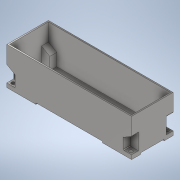
# Autodesk Inventor part: МПСТ Корпус
Saved by Autodesk Inventor 2022.1 (Build 261234020, 234B)
## iProperties
Created: 2021-11-18
Part Number: МПСТ Корпус
Material: Сталь, углеродистая
Document SubType Name: Modeling
Designer: Алексанян Г.
Density: 7.85 g/cm^3
Appearance: С умеренной полировкой
Author: Алексанян Г.
Autodesk Inventor part; units mm, degrees
ref_plane "YZ Plane" through (0, 0, 0) normal (1, 0, 0) x (0, 1, 0)
ref_plane "XZ Plane" through (0, 0, 0) normal (0, 1, 0) x (-1, 0, 0)
ref_plane "XY Plane" through (0, 0, 0) normal (0, 0, 1) x (1, 0, 0)
sketch "Эскиз1" plane through (0, 0, 0) normal (0, 1, 0) x (-1, 0, 0)
  line L0 (450, -150) -> (-450, -150)
  line L1 (-450, -150) -> (-450, 150)
  line L2 (-450, 150) -> (450, 150)
  line L3 (450, 150) -> (450, -150)
  line L4 (450, -150) -> (-450, 150) construction
  line L5 (-450, -150) -> (450, 150) construction
  point P0 (0, 0)
  dimension "d0" = 900
  dimension "d1" = 300
  constraints: 12 end point, 2 midpoint, 2 parallel, 1 horizontal, 1 perpendicular
  measures "d0" distance of L1.end L2.end
  measures "d1" distance of L0.end L1.end
extrude "Выдавливание1" add sketch "Эскиз1" against normal blind 270
sketch "Эскиз2" plane through (-450, 0, 150) normal (0, 0, 1) x (1, 0, 0)
  line L0 (210, -260) -> (690, -260)
  line L1 (690, -260) -> (690, -280)
  line L2 (690, -280) -> (210, -280)
  line L3 (210, -280) -> (210, -260)
  line L4 (900, -270) -> (0, -270) projected
  line L5 (210, -260) -> (690, -280) construction
  line L6 (690, -260) -> (210, -280) construction
  point P0 (450, 0)
  point P1 (450, -270)
  dimension "d4" = 480
  dimension "d5" = 20
  constraints: 12 end point, 3 midpoint, 2 parallel, 1 horizontal, 1 perpendicular
  measures "d4" distance of L1.end L2.end
  measures "d5" distance of L0.end L1.end
extrude "Выдавливание2" cut sketch "Эскиз2" against normal through all
sketch "Эскиз3" plane through (450, 0, 150) normal (1, 0, 0) x (0, 0, -1)
  line L0 (65, -260) -> (235, -260)
  line L1 (235, -260) -> (235, -280)
  line L2 (235, -280) -> (65, -280)
  line L3 (65, -280) -> (65, -260)
  line L4 (0, -270) -> (300, -270) projected
  line L5 (65, -260) -> (235, -280) construction
  line L6 (235, -260) -> (65, -280) construction
  point P0 (150, 0)
  point P1 (150, -270)
  dimension "d8" = 170
  dimension "d9" = 20
  constraints: 12 end point, 3 midpoint, 2 parallel, 1 horizontal, 1 perpendicular
  measures "d8" distance of L1.end L2.end
  measures "d9" distance of L0.end L1.end
extrude "Выдавливание3" cut sketch "Эскиз3" against normal through all
sketch "Эскиз4" plane through (-450, 0, 150) normal (0, 0, 1) x (1, 0, 0)
  line L0 (900, 0) -> (900, -270) projected
  line L1 (900, -240) -> (840, -240)
  line L2 (840, -240) -> (840, -160)
  line L3 (900, -110) -> (900, -240)
  line L4 (840, -160) -> (900, -125.359)
  line L5 (840, -160) -> (909.282, -160) construction
  line L6 (900, -270) -> (690, -270) projected
  point P0 (450, 0)
  point P1 (870, -240)
  dimension "d12" = 30
  dimension "d13" = 30
  dimension "d14" = 60
  dimension "d15" = 80
  constraints: 10 end point, 2 horizontal, 2 point on line, 1 equal length, 1 midpoint, 1 parallel, 1 perpendicular
  measures "d12" angle of L5 L4
  measures "d13" distance from line of L6 point (870, -240)
  measures "d14" distance between parallel lines of L2 L0
  measures "d15" distance from line of L1 L2.end
extrude "Выдавливание4" cut sketch "Эскиз4" against normal blind 50
sketch "Эскиз5" plane through (390, -240, 150) normal (0, 1, 0) x (1, 0, 0)
  line L0 (60, 50) -> (60, 0) projected
  line L1 (60, 0) -> (0, 0) projected
  point P0 (-390, 150)
  point P1 (35, 20)
  dimension "d18" = 25
  dimension "d19" = 20
  measures "d18" distance from line of L0 point (35, 20)
  measures "d19" distance from line of L1 point (35, 20)
hole "Отверстие1" at (425, -240, 130) direction (0, -1, 0) diameter 25 end through all
mirror "Зеркальное отражение1" about plane through (0, 0, 0) normal (1, 0, 0) of "Выдавливание4", "Отверстие1"
mirror "Зеркальное отражение2" about plane through (0, 0, 0) normal (0, 0, 1) of "Выдавливание4", "Отверстие1", "Зеркальное отражение1"
sketch "Эскиз6" plane through (0, 0, 0) normal (0, 1, 0) x (1, 0, 0)
  line L0 (-450, -150) -> (450, -150) construction
  line L1 (450, -150) -> (450, 150) construction
  line L2 (450, 150) -> (-450, 150) construction
  line L3 (-450, 150) -> (-450, -150) construction
  line L4 (-440, 140) -> (440, 140)
  line L5 (440, 140) -> (440, -140)
  line L6 (440, -140) -> (-440, -140)
  line L7 (-440, -140) -> (-440, 140)
  point P0 (0, 0)
  dimension "d27" = 10
  constraints: 8 end point, 3 other
  measures "d27" distance between parallel lines of L2 L4
extrude "Выдавливание5" cut sketch "Эскиз6" against normal up to surface (125.359 mm away)
sketch "Эскиз7" plane through (440, 0, 140) normal (0, 0, -1) x (-1, 0, 0)
  line L0 (50, -160) -> (-10, -125.359) construction
  line L1 (880, -125.359) -> (0, -125.359) projected
  line L2 (0, -125.359) -> (60, -160)
  line L3 (50, -160) -> (50, -240) projected
  line L4 (440, 70.8163) -> (440, -268.4276) construction
  line L5 (880, -125.359) -> (820, -160)
  line L6 (830, -240) -> (830, -160) projected
  line L7 (820, -160) -> (60, -160)
  point P0 (440, 0)
  dimension "d30" = 10
  dimension "d31" = 10
  constraints: 8 end point, 1 horizontal, 1 parallel, 1 symmetric about line, 1 vertical
  measures "d30" distance of L0.start L2.end
  measures "d31" distance from line of L6 L5.end
extrude "Выдавливание6" cut sketch "Эскиз7" along normal up to surface (280 mm away)
sketch "Эскиз8" plane through (-380, -160, 140) normal (0, 1, 0) x (1, 0, 0)
  line L0 (0, 280) -> (760, 280) construction
  line L1 (0, 0) -> (0, 280) construction
  line L2 (760, 0) -> (0, 0) construction
  line L3 (760, 0) -> (760, 280) construction
  line L4 (820, 50) -> (820, 230)
  line L5 (760, 0) -> (760, 280) projected
  line L6 (0, 280) -> (760, 280) projected
  line L7 (760, 280) -> (0, 280)
  line L8 (0, 0) -> (0, 280) projected
  line L9 (820, 50) -> (760, 50)
  line L10 (760, 50) -> (760, 0)
  line L11 (760, 0) -> (0, 0) projected
  line L12 (760, 0) -> (0, 0)
  line L13 (0, 0) -> (0, 50)
  line L14 (0, 50) -> (-60, 50)
  line L15 (-60, 50) -> (-60, 230)
  line L16 (380, -84.6684) -> (380, 409.964) construction
  line L17 (820, 230) -> (760, 230)
  line L18 (760, 230) -> (760, 280)
  line L19 (-60, 230) -> (0, 230)
  line L20 (0, 280) -> (0, 230)
  line L21 (-70, 40) -> (-10, 40) projected
  line L22 (-70, 225) -> (-70, 55) projected
  line L23 (-70, 240) -> (-10, 240) projected
  point P0 (380, 140)
  dimension "d37" = 10
  dimension "d38" = 10
  dimension "d39" = 10
  constraints: 26 end point, 7 point on line, 4 collinear, 4 perpendicular, 1 horizontal, 1 vertical, 3 other
  measures "d37" distance between parallel lines of L14 L21
  measures "d38" distance between parallel lines of L22 L15
  measures "d39" distance between parallel lines of L23 L19
extrude "Выдавливание7" cut sketch "Эскиз8" along normal mid plane 180
fillet "Сопряжение1" radius 5 20 edges at (-390, -160, 125) (-240, -260, 117.5) (-240, -260, -117.5) (240, -260, 117.5) (240, -260, -117.5) (390, -160, 125) (390, -160, -125) (-390, -160, -125) (345, -260, -85) (-345, -260, -85) (-345, -260, 85) (345, -260, 85) (450, -125.359, 125) (450, -125.359, -125) (-450, -125.359, -125) (-450, -125.359, 125) (-390, -240, 125) (390, -240, 125) (390, -240, -125) (-390, -240, -125)
equation "\"d38\" = d37"
equation "\"d39\" = d38"
